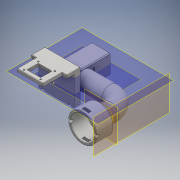
# Autodesk Inventor part: base2
Saved by Autodesk Inventor 2016 (Build 200138000, 138)
## iProperties
Created: 2016-02-15
Part Number: base2
Material: 一般
Document SubType Name: Modeling
Designer: Shun Hasegawa
Density: 1 g/cm^3
Appearance: 既定
Mass: 173.613 g
Surface Area: 764.814 cm^2
Volume: 173.613 cm^3
Author: Shun Hasegawa
Autodesk Inventor part; units mm, degrees
ref_plane "XZ Plane" through (0, 0, 0) normal (0, 1, 0) x (-1, 0, 0)
ref_plane "XY Plane" through (0, 0, 0) normal (0, 0, 1) x (1, 0, 0)
sketch "スケッチ1" plane through (0, 0, 0) normal (0, 1, 0) x (-1, 0, 0)
  line L0 (-25.5, -30) -> (25.5, -30)
  arc A0 (31.5, -30) -> (25.5, -30) centre (28.5, -30) ccw
  line L1 (31.5, -30) -> (36.5, -30)
  arc A1 (36.5, -30) -> (37.5, -29) centre (36.5, -29) ccw
  line L2 (37.5, -29) -> (37.5, 32)
  line L3 (37.5, 32) -> (-37.5, 32)
  line L4 (-37.5, 32) -> (-37.5, -29)
  arc A2 (-37.5, -29) -> (-36.5, -30) centre (-36.5, -29) ccw
  line L5 (-36.5, -30) -> (-31.5, -30)
  arc A3 (-25.5, -30) -> (-31.5, -30) centre (-28.5, -30) ccw
  circle A4 centre (13.5, 20) radius 2
  circle A5 centre (-13.5, 20) radius 2
  line L6 (0, -42.6485) -> (0, 44.4414) projected
  line L7 (-157.5414, 0) -> (70.2485, 0) projected
  point P0 (0, 0)
  dimension "d131" = 75
  dimension "d134" = 3
  dimension "d135" = 51
  dimension "d136" = 1
  dimension "d137" = 4
  dimension "d138" = 27
  dimension "d139" = 12
  dimension "d141" = 5
  dimension "d188" = 30
  dimension "d189" = 32
  constraints: 12 end point, 8 point on circle, 7 tangent, 6 centre point, 3 equal radius, 2 collinear, 2 perpendicular, 1 parallel, 1 symmetric about line, 1 other
  measures "d131" distance between parallel lines of L4 L2
  measures "d134" radius of A0
  measures "d135" distance of L0.start L0.end
  measures "d136" radius of A1
  measures "d137" diameter of A4
  measures "d138" distance of A5.centre A4.centre
  measures "d139" distance from line of A4.centre L3
  measures "d141" distance of L1.start L1.end
  measures "d188" distance between parallel lines of L0 L7
  measures "d189" distance between parallel lines of L7 L3
extrude "押し出し1" add sketch "スケッチ1" along normal blind 13
fillet "フィレット1" radius 1 6 edges at (-37.2071, 13, -29.7071) (-34, 13, -30) (-37.5, 13, 1.5) (37.2071, 13, -29.7071) (34, 13, -30) (37.5, 13, 1.5)
fillet "フィレット2" radius 1 1 edges at (0, 13, -30)
sketch "スケッチ2" plane through (0, 13, 0) normal (0, 1, 0) x (1, 0, 0)
  circle A0 centre (13.5, -20) radius 2 projected
  circle A1 centre (13.5, -20) radius 5
  circle A2 centre (-13.5, -20) radius 2 projected
  circle A3 centre (-13.5, -20) radius 5
  point P0 (0, 0)
  dimension "d4" = 10
  dimension "d5" = 10
  constraints: 2 centre point, 2 coincident
  measures "d4" diameter of A1
  measures "d5" diameter of A3
extrude "押し出し2" cut sketch "スケッチ2" against normal blind 4 contours A1
extrude "押し出し3" cut sketch "スケッチ2" against normal blind 4 contours A3
sketch "スケッチ3" plane through (0, 13, 0) normal (0, 1, 0) x (1, 0, 0)
  arc A0 (0, 0) -> (31.5, 30) centre (28.5, 30) ccw projected
  circle A1 centre (28.5, 30) radius 6.5
  arc A2 (-31.5, 30) -> (-25.5, 30) centre (-28.5, 30) ccw projected
  circle A3 centre (-28.5, 30) radius 6.5
  dimension "d10" = 13
  dimension "d11" = 13
  constraints: 2 centre point, 2 coincident, 1 other
  measures "d10" diameter of A1
  measures "d11" diameter of A3
extrude "押し出し4" cut sketch "スケッチ3" against normal blind 7 contours A1
extrude "押し出し5" cut sketch "スケッチ3" against normal blind 7 contours A3
sketch "スケッチ4" plane through (0, 13, 0) normal (0, 1, 0) x (1, 0, 0)
  line L0 (-20, -15) -> (20, -15)
  line L1 (20, -15) -> (20, 25)
  line L2 (20, 25) -> (-20, 25)
  line L3 (-20, 25) -> (-20, -15)
  line L4 (22, 30) -> (-22, 30) projected
  line L5 (-37.5, 29) -> (-37.5, -32) projected
  point P0 (0, 0)
  point P1 (-37.5, -10)
  dimension "d16" = 40
  dimension "d17" = 40
  dimension "d18" = 5
  dimension "d19" = 17.5
  constraints: 8 end point, 2 parallel, 1 horizontal, 1 perpendicular
  measures "d16" distance of L2.end L0.start
  measures "d17" distance of L1.end L2.end
  measures "d18" distance between parallel lines of L4 L2
  measures "d19" distance between parallel lines of L5 L3
extrude "押し出し6" add sketch "スケッチ4" along normal blind 80
sketch "スケッチ5" plane through (20, 13, 15) normal (1, 0, 0) x (0, 0, -1)
  circle A0 centre (20, 25) radius 18
  line L0 (44, 0) -> (-17, 0) projected
  line L1 (0, 0) -> (0, 80) projected
  point P0 (15, -13)
  point P1 (5, 0)
  point P2 (-14, 0)
  dimension "d22" = 36
  dimension "d23" = 25
  dimension "d26" = 20
  constraints: 1 centre point
  measures "d22" diameter of A0
  measures "d23" distance from line of L0 A0.centre
  measures "d26" distance from line of A0.centre L1
extrude "押し出し7" add sketch "スケッチ5" along normal blind 55
fillet "フィレット3" radius 2 4 edges at (20, 53, 15) (-20, 53, 15) (20, 53, -25) (-20, 53, -25)
sketch "スケッチ6" plane through (0, 93, 0) normal (0, 1, 0) x (1, 0, 0)
  line L0 (-14, -11) -> (14, -11)
  line L1 (16, -9) -> (16, 19)
  line L2 (14, 21) -> (-14, 21)
  line L3 (-16, 19) -> (-16, -9)
  line L4 (-20, 23) -> (-20, -13) projected
  line L5 (18, 25) -> (-18, 25) projected
  line L6 (-18, -15) -> (18, -15) projected
  line L7 (20, -13) -> (20, 23) projected
  arc A0 (-16, -9) -> (-14, -11) centre (-14, -9) ccw
  arc A1 (-14, 21) -> (-16, 19) centre (-14, 19) ccw
  arc A2 (16, 19) -> (14, 21) centre (14, 19) ccw
  arc A3 (14, -11) -> (16, -9) centre (14, -9) ccw
  point P0 (0, 0)
  dimension "d28" = 4
  dimension "d29" = 4
  dimension "d30" = 4
  dimension "d31" = 4
  dimension "d32" = 2
  constraints: 8 end point, 8 point on circle, 8 tangent, 4 centre point, 3 equal radius, 2 parallel, 1 horizontal, 1 perpendicular
  measures "d28" distance between parallel lines of L3 L4
  measures "d29" distance between parallel lines of L5 L2
  measures "d30" distance between parallel lines of L6 L0
  measures "d31" distance between parallel lines of L7 L1
  measures "d32" radius of A0
extrude "押し出し8" cut sketch "スケッチ6" against normal blind 90
sketch "スケッチ7" plane through (75, 38, -5) normal (1, 0, 0) x (0, 0, -1)
  arc A0 (18, 0) -> (-18, 0) centre (0, 0) ccw projected
  circle A1 centre (0, 0) radius 14
  point P0 (-5, -38)
  dimension "d35" = 4
  constraints: 1 centre point, 1 coincident
  measures "d35" radial gap between concentric circles of A1 A0
extrude "押し出し9" cut sketch "スケッチ7" against normal up to surface (59 mm away)
sketch "スケッチ9" plane through (75, 38, -5) normal (1, 0, 0) x (0, 0, -1)
  circle A0 centre (0, 0) radius 14 projected
  circle A1 centre (0, 0) radius 18 projected
  point P0 (-5, -38)
ref_plane "作業平面1" through (75, 38, -5) normal (0, 0, -1) x (-1, 0, 0)
sketch "スケッチ10" plane through (75, 38, -5) normal (0, 0, -1) x (-1, 0, 0)
  line L0 (55, -18) -> (0, -18) projected
  line L1 (0, -14) -> (0, 14) projected
  arc A0 (0, 0) -> (-32, -32) centre (0, -32) ccw
  line L2 (0, -32) -> (-32, -32) construction
  line L3 (0, -32) -> (0, 0) construction
  point P0 (75, -38)
  dimension "d39" = 14
  dimension "d40" = 90
  constraints: 4 end point, 2 point on circle, 1 centre point, 1 coincident, 1 midpoint, 1 point on line
  measures "d39" distance from line of point (0, -32) L0
  measures "d40" angle of L3 L2
sweep "スイープ1" add profiles "スケッチ9" path "スケッチ10" path curves A0
sketch "スケッチ11" plane through (107, 6, -5) normal (0, -1, 0) x (1, 0, 0)
  circle A0 centre (0, 0) radius 14 projected
  circle A1 centre (0, 0) radius 18 projected
  point P0 (-107, 5)
extrude "押し出し10" add sketch "スケッチ11" along normal blind 12
sketch "スケッチ12" plane through (107, -6, -5) normal (0, -1, 0) x (1, 0, 0)
  circle A0 centre (0, 0) radius 18 projected
  point P0 (-107, 5)
ref_plane "作業平面2" through (107, -18, -5) normal (0, -1, 0) x (1, 0, 0)
sketch "スケッチ13" plane through (107, -18, -5) normal (0, -1, 0) x (1, 0, 0)
  circle A0 centre (0, 0) radius 30
  point P0 (-107, 5)
  dimension "d46" = 60
  constraints: 1 centre point
  measures "d46" diameter of A0
loft "ロフト1" add profiles "スケッチ13" section 1 edges at (89, -6, -5)
ref_plane "作業平面3" through (107, -13, -5) normal (0, -1, 0) x (1, 0, 0)
sketch "スケッチ15" plane through (107, -13, -5) normal (0, -1, 0) x (1, 0, 0)
  circle A0 centre (0, 0) radius 19.25
  point P0 (-107, 5)
  dimension "d53" = 38.5
  constraints: 1 centre point, 1 coincident
  measures "d53" diameter of A0
sketch "スケッチ18" plane through (107, -18, -5) normal (0, -1, 0) x (1, 0, 0)
  circle A0 centre (0, 0) radius 25
  point P0 (-107, 5)
  dimension "d56" = 50
  constraints: 1 centre point, 1 coincident
  measures "d56" diameter of A0
loft "ロフト2" cut profiles "スケッチ18", "スケッチ15"
sketch "スケッチ19" plane through (107, -13, -5) normal (0, -1, 0) x (1, 0, 0)
  circle A0 centre (0, 0) radius 14
  point P0 (-107, 5)
  dimension "d61" = 28
  constraints: 1 centre point, 1 coincident
  measures "d61" diameter of A0
extrude "押し出し11" cut sketch "スケッチ19" against normal blind 7
sketch "スケッチ20" plane through (107, -18, -5) normal (0, -1, 0) x (1, 0, 0)
  circle A0 centre (0, 0) radius 25 projected
  circle A1 centre (0, 0) radius 30 projected
  point P0 (-107, 5)
extrude "押し出し12" add sketch "スケッチ20" along normal blind 34.5
fillet "フィレット4" radius 1 1 edges at (77, -52.5, -5)
fillet "フィレット5" radius 1 1 edges at (82, -52.5, -5)
ref_plane "作業平面4" through (107, -18, 25) normal (0, 0, -1) x (-1, 0, 0)
sketch "スケッチ21" plane through (107, -18, 25) normal (0, 0, -1) x (-1, 0, 0)
  line L0 (6, -24) -> (-8, -24)
  line L1 (-8, -24) -> (-8, -30)
  line L2 (-8, -30) -> (6, -30)
  line L3 (6, -30) -> (6, -24)
  line L4 (29, -34.5) -> (-29, -34.5) projected
  line L5 (30, 0) -> (30, -33.5) projected
  point P0 (107, 18)
  dimension "d68" = 4.5
  dimension "d69" = 6
  dimension "d70" = 14
  dimension "d71" = 24
  constraints: 8 end point, 2 parallel, 1 horizontal, 1 perpendicular
  measures "d68" distance between parallel lines of L4 L2
  measures "d69" distance of L2.end L0.start
  measures "d70" distance of L0.start L0.end
  measures "d71" distance between parallel lines of L3 L5
extrude "押し出し13" cut sketch "スケッチ21" along normal through all
ref_plane "作業平面5" through (137, -18, -5) normal (1, 0, 0) x (0, 1, 0)
sketch "スケッチ22" plane through (137, -18, -5) normal (1, 0, 0) x (0, 1, 0)
  line L0 (-34.5, -29) -> (-34.5, 29) projected
  line L1 (-34.5, 2) -> (-32, 2)
  line L2 (-32, -4) -> (-34.5, -4)
  line L3 (-34.5, -4) -> (-34.5, 2)
  arc A0 (-32, -4) -> (-32, 2) centre (-32, -1) ccw
  point P0 (18, 5)
  dimension "d76" = 6
  dimension "d77" = 2.5
  dimension "d78" = 3
  dimension "d79" = 3
  dimension "d80" = 30
  constraints: 6 end point, 2 point on circle, 1 centre point, 1 horizontal, 1 parallel, 1 point on line
  measures "d76" distance between parallel lines of L2 L1
  measures "d77" distance of L1.start L1.end
  measures "d78" radius of A0
  measures "d79" distance from line of A0.centre L1
  measures "d80" vertical distance of A0.centre L0.end
extrude "押し出し14" cut sketch "スケッチ22" against normal through all
sketch "スケッチ23" plane through (107, -13, -5) normal (0, -1, 0) x (1, 0, 0)
  circle A0 centre (0, 0) radius 16
  circle A1 centre (0, 0) radius 17.5
  point P0 (-107, 5)
  dimension "d83" = 32
  dimension "d84" = 35
  constraints: 2 centre point, 1 coincident
  measures "d83" diameter of A0
  measures "d84" diameter of A1
extrude "押し出し15" add sketch "スケッチ23" along normal blind 3
fillet "フィレット6" radius 0.75 1 edges at (91, -16, -5)
fillet "フィレット7" radius 0.75 1 edges at (89.5, -16, -5)
sketch "スケッチ27" plane through (20, 38, -23) normal (1, 0, 0) x (0, 0, -1)
  circle A0 centre (-25.62, 28.5) radius 1.4
  circle A1 centre (-10.38, 28.5) radius 1.4
  line L0 (-27.5, 19) -> (-8.5, 19)
  line L1 (-7.5, 20) -> (-7.5, 22)
  line L2 (-8.5, 23) -> (-27.5, 23)
  line L3 (-28.5, 22) -> (-28.5, 20)
  line L4 (-36, 55) -> (0, 55) projected
  arc A2 (-28.5, 20) -> (-27.5, 19) centre (-27.5, 20) ccw
  arc A3 (-8.5, 19) -> (-7.5, 20) centre (-8.5, 20) ccw
  arc A4 (-7.5, 22) -> (-8.5, 23) centre (-8.5, 22) ccw
  arc A5 (-27.5, 23) -> (-28.5, 22) centre (-27.5, 22) ccw
  line L5 (-38, 55) -> (-38, -25) projected
  line L6 (2, -25) -> (2, 55) projected
  point P0 (-23, -38)
  dimension "d116" = 36
  dimension "d117" = 2.8
  dimension "d119" = 1
  dimension "d120" = 21
  dimension "d121" = 4
  dimension "d122" = 2.8
  dimension "d123" = 9.5
  dimension "d124" = 15.24
  dimension "d125" = 2.88
  dimension "d126" = 2.88
  dimension "d127" = 9.5
  dimension "d128" = 9.5
  constraints: 8 end point, 8 point on circle, 8 tangent, 6 centre point, 3 equal radius, 2 parallel, 1 horizontal, 1 horizontal alignment, 1 perpendicular
  measures "d116" distance between parallel lines of L0 L4
  measures "d117" diameter of A0
  measures "d119" radius of A2
  measures "d120" distance between parallel lines of L1 L3
  measures "d121" distance between parallel lines of L2 L0
  measures "d122" diameter of A1
  measures "d123" distance from line of L0 A0.centre
  measures "d124" distance of A1.centre A0.centre
  measures "d125" distance from line of A1.centre L1
  measures "d126" distance from line of A0.centre L3
  measures "d127" distance between parallel lines of L3 L5
  measures "d128" distance between parallel lines of L6 L1
extrude "押し出し20" cut sketch "スケッチ27" against normal up to next
sketch "スケッチ28" plane through (-37.5, 0, 32) normal (0, 0, 1) x (1, 0, 0)
  line L0 (0, 13) -> (75, 13)
  line L1 (75, 13) -> (75, -56)
  line L2 (75, -56) -> (0, -56)
  line L3 (0, -56) -> (0, 13)
  line L4 (1, 13) -> (74, 13) projected
  line L5 (75, 0) -> (75, 12) projected
  line L6 (0, 0) -> (0, 12) projected
  point P0 (37.5, 0)
  dimension "d143" = 69
  constraints: 8 end point, 3 point on line, 2 parallel, 1 horizontal, 1 perpendicular
  measures "d143" distance between parallel lines of L0 L2
extrude "押し出し21" add sketch "スケッチ28" along normal blind 6
fillet "フィレット8" radius 1 2 edges at (-37.5, 13, 35) (37.5, 13, 35)
fillet "フィレット9" radius 1 5 edges at (-37.2071, 12.7071, 38) (-37.5, -22, 38) (37.2071, 12.7071, 38) (37.5, -21.9999, 38) (0, 13, 38)
sketch "スケッチ32" plane through (-37.5, 0, 38) normal (0, 0, 1) x (1, 0, 0)
  circle A0 centre (20, -21) radius 1.6
  circle A1 centre (55, -21) radius 1.6
  circle A2 centre (20, -51) radius 1.6
  circle A3 centre (55, -51) radius 1.6
  line L0 (1, -56) -> (74, -56) projected
  line L1 (1, -56) -> (1, 12) projected
  line L2 (74, 12) -> (74, -56) projected
  point P0 (37.5, 0)
  dimension "d165" = 3.2
  dimension "d166" = 35
  dimension "d167" = 35
  dimension "d168" = 19
  dimension "d169" = 19
  dimension "d170" = 5
  constraints: 4 centre point, 3 equal radius, 2 horizontal alignment, 2 vertical alignment
  measures "d165" diameter of A2
  measures "d166" distance from line of A0.centre L0
  measures "d167" distance of A1.centre A0.centre
  measures "d168" distance from line of A0.centre L1
  measures "d169" distance from line of L2 A1.centre
  measures "d170" distance from line of L0 A2.centre
extrude "押し出し25" cut sketch "スケッチ32" against normal up to next
sketch "スケッチ33" plane through (-37.5, 0, 32) normal (0, 0, -1) x (-1, 0, 0)
  circle A0 centre (-20, -21) radius 1.6 projected
  circle A1 centre (-20, -21) radius 3
  circle A2 centre (-20, -51) radius 1.6 projected
  circle A3 centre (-20, -51) radius 3
  circle A4 centre (-55, -21) radius 1.6 projected
  circle A5 centre (-55, -21) radius 3
  circle A6 centre (-55, -51) radius 1.6 projected
  circle A7 centre (-55, -51) radius 3
  point P0 (-37.5, 0)
  dimension "d173" = 6
  constraints: 4 centre point, 4 coincident, 3 equal radius
  measures "d173" diameter of A1
extrude "押し出し26" cut sketch "スケッチ33" against normal blind 2.5
sketch "スケッチ34" plane through (-37.5, 0, 38) normal (0, 0, 1) x (1, 0, 0)
  line L0 (25, -24) -> (50, -24)
  line L1 (52, -26) -> (52, -46)
  line L2 (50, -48) -> (25, -48)
  line L3 (23, -46) -> (23, -26)
  arc A0 (25, -24) -> (23, -26) centre (25, -26) ccw
  arc A1 (23, -46) -> (25, -48) centre (25, -46) ccw
  arc A2 (50, -48) -> (52, -46) centre (50, -46) ccw
  arc A3 (52, -26) -> (50, -24) centre (50, -26) ccw
  circle A4 centre (55, -21) radius 1.6 projected
  circle A5 centre (20, -51) radius 1.6 projected
  point P0 (37.5, 0)
  dimension "d176" = 2
  dimension "d177" = 3
  dimension "d178" = 3
  dimension "d179" = 3
  dimension "d180" = 3
  constraints: 8 end point, 8 point on circle, 8 tangent, 4 centre point, 3 equal radius, 2 parallel, 1 horizontal, 1 perpendicular
  measures "d176" radius of A0
  measures "d177" distance from line of L0 A4.centre
  measures "d178" distance from line of A5.centre L2
  measures "d179" distance from line of A5.centre L3
  measures "d180" distance from line of A4.centre L1
extrude "押し出し27" cut sketch "スケッチ34" against normal up to next contours L0 A3 L1 A2 L2 A1 L3 A0
sketch "スケッチ35" plane through (-37.5, 0, 32) normal (0, 0, -1) x (-1, 0, 0)
  line L0 (0, 12) -> (0, -56) projected
  line L1 (0, -56) -> (-10, -56)
  line L2 (-10, -56) -> (-10, -16)
  line L3 (-10, -16) -> (0, -16)
  line L4 (0, -16) -> (0, -56)
  line L5 (-75, 0) -> (-75, -56) projected
  line L6 (-75, -56) -> (-65, -56)
  line L7 (-65, -56) -> (-65, -16)
  line L8 (-65, -16) -> (-75, -16)
  line L9 (-75, -16) -> (-75, -56)
  point P0 (-37.5, 0)
  dimension "d183" = 10
  dimension "d184" = 40
  constraints: 16 end point, 4 parallel, 2 equal length, 2 horizontal, 2 perpendicular
  measures "d183" distance of L0.end L1.end
  measures "d184" distance of L1.end L2.end
extrude "押し出し28" cut sketch "スケッチ35" against normal up to next
fillet "フィレット10" radius 1 11 edges at (-27.5, -36, 38) (0, -56, 38) (27.5, -36, 38) (37.2071, -16, 37.7071) (37.5, -16, 34.5) (32, -16, 38) (-37.2071, -16, 37.7071) (-37.5, -16, 34.5) (-32, -16, 38) (-27.5, -56, 35) (27.5, -56, 35)
fillet "フィレット11" radius 2 1 edges at (0, 0, 32)
